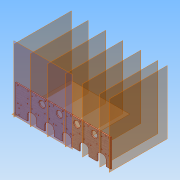
# Autodesk Inventor part: Pancake_Top Board
Saved by Autodesk Inventor 2018.1 (Build 221171000, 171)
## iProperties
Created: 2019-02-21
Part Number: Pancake_Top Board
Material: Wood (Oak)
Document SubType Name: Modeling
Designer: James
Density: 0.76 g/cm^3
Appearance: White Oak - Natural Medium Gloss
Author: James
Autodesk Inventor part; units mm, degrees
ref_plane "YZ Plane" through (0, 0, 0) normal (1, 0, 0) x (0, 1, 0)
ref_plane "XZ Plane" through (0, 0, 0) normal (0, 1, 0) x (-1, 0, 0)
ref_plane "XY Plane" through (0, 0, 0) normal (0, 0, 1) x (1, 0, 0)
derived "Pancake_Skeleton.ipt"
ref_plane "Ground" through (0, 0, 0) normal (0, 1, 0) x (-1, 0, 0)
ref_plane "Back" through (0, 0, 0) normal (0, 0, 1) x (1, 0, 0)
ref_plane "LHS" through (0, 0, 0) normal (1, 0, 0) x (0, 1, 0)
ref_plane "Lane 1" through (90, 0, 0) normal (1, 0, 0) x (0, 1, 0)
ref_plane "Lane 2" through (185, 0, 0) normal (1, 0, 0) x (0, 1, 0)
ref_plane "Lane 3" through (280, 0, 0) normal (1, 0, 0) x (0, 1, 0)
ref_plane "Lane 4" through (375, 0, 0) normal (1, 0, 0) x (0, 1, 0)
ref_plane "Lane 5" through (470, 0, 0) normal (1, 0, 0) x (0, 1, 0)
ref_plane "RHS" through (520, 0, 0) normal (1, 0, 0) x (0, 1, 0)
sketch "Sketch1" plane through (0, 0, 0) normal (0, 1, 0) x (-1, 0, 0)
  line L0 (-624, 0) -> (104, 0) projected
  line L1 (0, -30) -> (0, 180) projected
  line L2 (0, 0) -> (-520, 0)
  line L3 (-520, 0) -> (-520, 150)
  line L4 (-520, 150) -> (0, 150)
  line L5 (0, 150) -> (0, 0)
  line L6 (-520, -30) -> (-520, 180) projected
  dimension "d1" = 150
  constraints: 8 end point, 2 parallel, 1 collinear, 1 horizontal, 1 perpendicular
  measures "d1" distance of L2.end L3.end
extrude "Extrusion1" add sketch "Sketch1" along normal blind 5
sketch "Sketch2" plane through (0, 5, 0) normal (0, 1, 0) x (1, 0, 0)
  line L0 (0, -150) -> (520, -150) projected
  line L1 (90, 30) -> (90, -180) projected
  line L2 (185, 30) -> (185, -180) projected
  point P0 (0, 0)
  point P1 (145, -120)
  dimension "d4" = 30
  dimension "d90" = 40
  measures "d4" distance from line of point (145, -120) L0
  measures "d90" distance from line of point (145, -120) L2
hole "Hole1" at (145, 5, 120) direction (0, -1, 0) diameter 35 end through all
pattern_linear "Rectangular Pattern1" count 4 spacing 95 along (1, 0, 0) of "Hole1"
sketch "Sketch3" plane through (0, 5, 0) normal (0, 1, 0) x (1, 0, 0)
  line L0 (0, 0) -> (0, -150) projected
  line L1 (624, 0) -> (-104, 0) projected
  line L2 (0, -150) -> (520, -150) projected
  point P0 (12.5, -57.5)
  point P1 (12.5, -142.5)
  dimension "d16" = 12.5
  dimension "d18" = 85
  dimension "d66" = 7.5
  constraints: 1 vertical alignment
  measures "d16" distance from line of L0 point (12.5, -57.5)
  measures "d18" distance of point (12.5, -142.5) point (12.5, -57.5)
  measures "d66" distance from line of L2 point (12.5, -142.5)
hole "Hole2" at (12.5, 5, 57.5) at (12.5, 5, 142.5) direction (0, -1, 0) diameter 4.5 end through all countersink diameter 9.4 countersink angle 90 clearance for "Flat Head Machine Screw" size "M4" standard "Ansi Metric M Profile"
ref_plane "Mid plane" through (260, 0, 0) normal (-1, 0, 0) x (0, 0, 1)
mirror "Mirror1" about plane through (260, 0, 0) normal (-1, 0, 0) of "Hole2"
sketch "Sketch4" plane through (0, 5, 0) normal (0, 1, 0) x (1, 0, 0)
  line L0 (624, 0) -> (-104, 0) projected
  line L1 (0, -150) -> (520, -150) projected
  line L2 (90, 30) -> (90, -180) projected
  point P0 (0, 0)
  point P1 (112, -57.5)
  point P2 (112, -142.5)
  dimension "d28" = 7.5
  dimension "d29" = 22
  dimension "d68" = 85
  constraints: 1 vertical alignment
  measures "d28" distance from line of L1 point (112, -142.5)
  measures "d29" distance from line of L2 point (112, -57.5)
  measures "d68" distance of point (112, -142.5) point (112, -57.5)
hole "Hole3" at (112, 5, 57.5) at (112, 5, 142.5) direction (0, -1, 0) diameter 4.5 end through all clearance for "Socket Head Cap Screw" size "M4" standard "Ansi Metric M Profile"
pattern_linear "Rectangular Pattern2" count 5 spacing 95 along (1, 0, 0) of "Hole3"
sketch "Sketch5" plane through (0, 5, 0) normal (0, 1, 0) x (1, 0, 0)
  line L0 (624, 0) -> (-104, 0) projected
  line L1 (90, 30) -> (90, -180) projected
  line L2 (0, -150) -> (520, -150) projected
  point P0 (0, 0)
  point P1 (30, -57.5)
  point P2 (65, -82.5)
  dimension "d41" = 57.5
  dimension "d42" = 60
  dimension "d78" = 25
  dimension "d79" = 35
  measures "d41" distance from line of L0 point (30, -57.5)
  measures "d42" distance from line of L1 point (30, -57.5)
  measures "d78" vertical distance of point (65, -82.5) point (30, -57.5)
  measures "d79" horizontal distance of point (65, -82.5) point (30, -57.5)
hole "Hole4" at (30, 5, 57.5) at (65, 5, 82.5) direction (0, -1, 0) diameter 4.5 end through all clearance for "Socket Head Cap Screw" size "M4" standard "Ansi Metric M Profile"
pattern_linear "Rectangular Pattern3" count 5 spacing 95 along (1, 0, 0) of "Hole4"
sketch "Sketch6" plane through (0, 5, 0) normal (0, 1, 0) x (1, 0, 0)
  line L0 (624, 0) -> (-104, 0) projected
  line L1 (90, 30) -> (90, -180) projected
  line L2 (0, -150) -> (520, -150) projected
  point P0 (0, 0)
  point P1 (90, -70)
  point P2 (90, -130)
  dimension "d53" = 60
  dimension "d67" = 20
  constraints: 1 point on line, 1 vertical alignment
  measures "d53" distance of point (90, -130) point (90, -70)
  measures "d67" distance from line of L2 point (90, -130)
hole "Hole5" at (90, 5, 70) at (90, 5, 130) direction (0, -1, 0) diameter 4.5 end through all countersink diameter 9.4 countersink angle 90 clearance for "Flat Head Machine Screw" size "M4" standard "Ansi Metric M Profile"
pattern_linear "Rectangular Pattern4" count 5 spacing 95 along (1, 0, 0) of "Hole5"
sketch "Sketch7" plane through (0, 5, 0) normal (0, 1, 0) x (1, 0, 0)
  line L0 (65, -50) -> (115, -50)
  line L1 (115, -50) -> (115, 0)
  line L2 (115, 0) -> (65, 0)
  line L3 (65, 0) -> (65, -50)
  line L4 (520, 0) -> (0, 0) projected
  line L5 (90, 30) -> (90, -180) projected
  dimension "d69" = 25
  dimension "d70" = 50
  dimension "d71" = 50
  constraints: 8 end point, 2 parallel, 1 collinear, 1 horizontal, 1 perpendicular
  measures "d69" distance between parallel lines of L5 L1
  measures "d70" distance of L0.start L0.end
  measures "d71" distance of L0.end L1.end
extrude "Extrusion2" cut sketch "Sketch7" against normal through all
fillet "Fillet1" radius 20 2 edges at (65, 2.5, 50) (115, 2.5, 50)
pattern_linear "Rectangular Pattern5" count 5 spacing 95 along (1, 0, 0) of "Extrusion2", "Fillet1"
sketch "Sketch8" plane through (0, 5, 0) normal (0, 1, 0) x (1, 0, 0)
  circle A0 centre (30, -57.5) radius 2.25 projected
  line L0 (624, 0) -> (-104, 0) projected
  point P0 (0, 0)
  point P1 (20, -37.5)
  point P2 (20, -7.5)
  dimension "d80" = 30
  dimension "d81" = 10
  dimension "d82" = 7.5
  constraints: 1 vertical alignment
  measures "d80" distance of point (20, -37.5) point (20, -7.5)
  measures "d81" horizontal distance of A0.centre point (20, -37.5)
  measures "d82" distance from line of L0 point (20, -7.5)
hole "Hole6" at (20, 5, 37.5) at (20, 5, 7.5) direction (0, -1, 0) diameter 4.5 end through all clearance for "Flat Head Machine Screw" size "M4" standard "Ansi Metric M Profile"
sketch "Sketch9" plane through (0, 5, 0) normal (0, 1, 0) x (1, 0, 0)
  line L0 (90, 30) -> (90, -180) projected
  line L1 (0, -150) -> (520, -150) projected
  point P0 (0, 0)
  point P1 (68, -107.5)
  point P2 (68, -142.5)
  dimension "d95" = 22
  dimension "d96" = 7.5
  dimension "d97" = 35
  constraints: 1 vertical alignment
  measures "d95" distance from line of L0 point (68, -142.5)
  measures "d96" distance from line of L1 point (68, -142.5)
  measures "d97" distance of point (68, -107.5) point (68, -142.5)
hole "Hole7" at (68, 5, 107.5) at (68, 5, 142.5) direction (0, -1, 0) diameter 4.5 end through all clearance for "Flat Head Machine Screw" size "M4" standard "Ansi Metric M Profile"
sketch "Sketch11" plane through (0, 0, 0) normal (0, -1, 0) x (1, 0, 0)
  line L0 (520, 150) -> (0, 150) projected
  line L1 (185, 180) -> (185, -30) projected
  point P0 (0, 0)
  point P1 (162, 142.5)
  dimension "d105" = 7.5
  dimension "d106" = 23
  measures "d105" distance from line of point (162, 142.5) L0
  measures "d106" distance from line of L1 point (162, 142.5)
hole "Hole8" at (162, 0, 142.5) direction (0, 1, 0) diameter 3.4 end through all countersink diameter 6.3 countersink angle 90 clearance for "Flat Head Machine Screw" size "M3" standard "Ansi Metric M Profile"
pattern_linear "Rectangular Pattern6" count 4 spacing 95 along (1, 0, 0) of "Hole8"
sketch "Sketch12" plane through (0, 0, 150) normal (0, 0, 1) x (1, 0, 0)
  line L0 (0, 5) -> (520, 5) projected
  line L1 (520, 0) -> (0, 0) projected
  line L2 (160.3, 5) -> (163.7, 5) projected
  line L3 (160.3, 5) -> (163.7, 5) projected
  line L4 (160.3, 1.45) -> (163.7, 1.45) projected
  line L5 (209.25, 0) -> (204.75, 0) projected
  line L6 (204.75, 5) -> (209.25, 5) projected
  line L7 (209.25, 0) -> (209.25, 5) projected
  line L8 (185, 6) -> (185, -1) projected
  point P0 (167, 2.5)
  point P1 (213, 2.5)
  dimension "d117" = 2.5
  dimension "d118" = 2.5
  dimension "d130" = 18
  dimension "d131" = 28
  constraints: 1 horizontal alignment
  measures "d117" distance from line of point (167, 2.5) L0
  measures "d118" distance from line of L1 point (167, 2.5)
  measures "d130" distance from line of L8 point (167, 2.5)
  measures "d131" distance from line of L8 point (213, 2.5)
hole "Hole9" at (167, 2.5, 150) at (213, 2.5, 150) direction (0, 0, -1) diameter 1.755 depth 6.353 tip angle 118 thread size "2-64 UNF" class "2B" standard "ANSI Unified Screw Threads"
pattern_linear "Rectangular Pattern7" count 3 spacing 95 along (1, 0, 0) of "Hole9"
equation "\"d69\" = 0.5 * d70"
equation "\"d117\" = d118"
body "Solid1"
